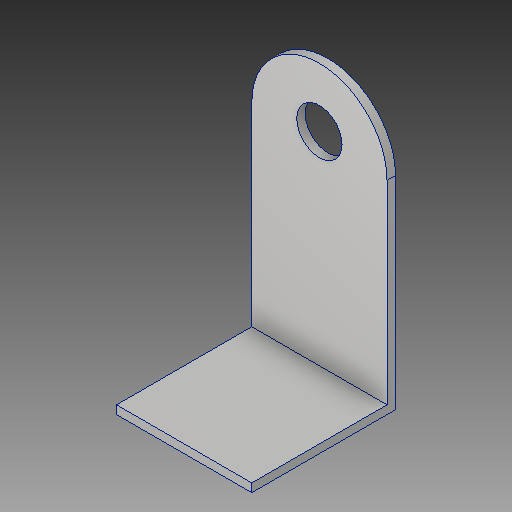
# Autodesk Inventor part: L Connector Ramp
Saved by Autodesk Inventor 2017 (Build 210142000, 142)
## iProperties
Created: 2018-01-20
Part Number: L Connector Ramp
Material: Aluminum 6061
Document SubType Name: Modeling
Designer: S346795925
Density: 2.7 g/cm^3
Appearance: Aluminum - Flat
Author: S346795925
Autodesk Inventor part; units mm, degrees
ref_plane "YZ Plane" through (0, 0, 0) normal (1, 0, 0) x (0, 1, 0)
ref_plane "XZ Plane" through (0, 0, 0) normal (0, 1, 0) x (-1, 0, 0)
ref_plane "XY Plane" through (0, 0, 0) normal (0, 0, 1) x (1, 0, 0)
sketch "Sketch1" plane through (0, 0, 0) normal (1, 0, 0) x (0, 1, 0)
  line L0 (0, 0) -> (-3.175, 0)
  line L1 (-3.175, 0) -> (-3.175, -50.8)
  line L2 (-3.175, -50.8) -> (0, -50.8)
  line L3 (0, -50.8) -> (0, 0)
  line L4 (-3.175, -50.8) -> (98.425, -50.8)
  line L5 (98.425, -50.8) -> (98.425, -53.975)
  line L6 (98.425, -53.975) -> (-3.175, -53.975)
  line L7 (-3.175, -53.975) -> (-3.175, -50.8)
  dimension "d0" = 3.175
  dimension "d1" = 50.8
  dimension "d2" = 101.6
  dimension "d3" = 3.175
  constraints: 16 end point, 4 parallel, 2 horizontal, 2 perpendicular
  measures "d0" distance of L2.end L1.end
  measures "d1" distance of L1.end L0.end
  measures "d2" distance of L5.end L6.end
  measures "d3" distance of L4.end L5.end
extrude "Extrusion1" add sketch "Sketch1" along normal blind 50.8
sketch "Sketch2" plane through (0, 0, -50.8) normal (0, 0, 1) x (1, 0, 0)
  circle A0 centre (25.4, 76.2) radius 8.509
  line L0 (0, 98.425) -> (0, 0) projected
  line L1 (0, 0) -> (50.8, 0) projected
  dimension "d6" = 17.018
  dimension "d7" = 25.4
  dimension "d8" = 76.2
  constraints: 1 centre point
  measures "d6" diameter of A0
  measures "d7" distance from line of L0 A0.centre
  measures "d8" distance from line of L1 A0.centre
extrude "Extrusion2" cut sketch "Sketch2" against normal through all
fillet "Fillet1" radius 25.4 2 edges at (50.8, 98.425, -52.3875) (0, 98.425, -52.3875)
body "Solid1"
